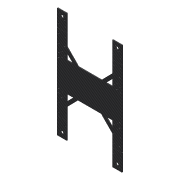
# Autodesk Inventor part: chassis mit motorlöcher
Saved by Autodesk Inventor 2018 (Build 220112000, 112)
## iProperties
Created: 2018-01-20
Part Number: chassis mit motorlöcher
Material: CFK
Document SubType Name: Modeling
Designer: fhinstall
Density: 1.43 g/cm^3
Appearance: Kohlenstofffaser
Mass: 133.015 g
Surface Area: 687.489 cm^2
Volume: 93.0173 cm^3
Author: fhinstall
Autodesk Inventor part; units mm, degrees
ref_plane "YZ Plane" through (0, 0, 0) normal (1, 0, 0) x (0, 1, 0)
ref_plane "XZ Plane" through (0, 0, 0) normal (0, 1, 0) x (-1, 0, 0)
ref_plane "XY Plane" through (0, 0, 0) normal (0, 0, 1) x (1, 0, 0)
sketch "Skizze1" plane through (0, 0, 0) normal (0, 1, 0) x (-1, 0, 0)
  line L0 (127.3199, 0) -> (-102.7808, 0) construction
  line L1 (0, 142.2638) -> (0, -235.5235) construction
  line L2 (100, 50) -> (100, 0)
  line L3 (70, 45) -> (0, 45)
  line L4 (0, 0) -> (100, 0)
  line L5 (0, 45) -> (0, 0)
  line L6 (100, 50) -> (100, 170)
  line L7 (100, 170) -> (70, 170)
  line L8 (70, 170) -> (70, 45)
  circle A0 centre (95, 41) radius 1.7
  line L9 (100, 140) -> (70, 140) construction
  circle A1 centre (85, 155) radius 4
  circle A2 centre (79.7789, 161.0614) radius 1.7
  circle A3 centre (92.1979, 161.2) radius 1.7
  circle A4 centre (90.2211, 148.9386) radius 1.7
  circle A5 centre (77.8021, 148.8) radius 1.7
  circle A6 centre (85, 155) radius 8 construction
  circle A7 centre (85, 155) radius 9.5 construction
  line L10 (79.7789, 161.0614) -> (90.2211, 148.9386) construction
  line L11 (92.1979, 161.2) -> (77.8021, 148.8) construction
  arc A8 (92.0223, 145.331) -> (96.9015, 153.9244) centre (85, 155) ccw construction
  line L12 (96.9015, 153.9244) -> (96.6242, 153.848) construction
  arc A9 (94.3917, 161.9459) -> (96.6242, 153.848) centre (95.508, 157.8969) ccw construction
  line L13 (94.3917, 161.9459) -> (94.669, 162.0223) construction
  arc A10 (94.669, 162.0223) -> (86.0756, 166.9015) centre (85, 155) ccw construction
  line L14 (86.0756, 166.9015) -> (86.152, 166.6242) construction
  arc A11 (78.0541, 164.3917) -> (86.152, 166.6242) centre (82.1031, 165.508) ccw construction
  line L15 (78.0541, 164.3917) -> (77.9777, 164.669) construction
  arc A12 (77.9777, 164.669) -> (73.0985, 156.0756) centre (85, 155) ccw construction
  line L16 (73.0985, 156.0756) -> (73.3758, 156.152) construction
  arc A13 (75.6083, 148.0541) -> (73.3758, 156.152) centre (74.492, 152.1031) ccw construction
  line L17 (75.6083, 148.0541) -> (75.331, 147.9777) construction
  arc A14 (75.331, 147.9777) -> (83.9244, 143.0985) centre (85, 155) ccw construction
  line L18 (83.9244, 143.0985) -> (83.848, 143.3758) construction
  arc A15 (91.9459, 145.6083) -> (83.848, 143.3758) centre (87.8969, 144.492) ccw construction
  line L19 (91.9459, 145.6083) -> (92.0223, 145.331) construction
  circle A16 centre (85, 155) radius 4 construction
  circle A17 centre (78.0432, 158.95) radius 1.25 construction
  circle A18 centre (89.6906, 163.2613) radius 1.25 construction
  circle A19 centre (91.9568, 151.05) radius 1.25 construction
  circle A20 centre (80.3094, 146.7387) radius 1.25 construction
  line L20 (70, 117.8095) -> (70, 117.3095)
  line L21 (100, 118) -> (70, 118)
  line L22 (70, 118) -> (70, 117.5)
  line L23 (70, 117.5) -> (100, 117.5)
  line L24 (100, 117.5) -> (100, 118)
  circle A21 centre (95.0005, 132.5) radius 1.7
  circle A22 centre (75.0005, 132.5) radius 1.7
  circle A23 centre (75, 105.2) radius 1.7
  circle A24 centre (95, 105.2) radius 1.7
  circle A25 centre (95, 79.2) radius 1.7
  circle A26 centre (75, 79.2) radius 1.7
  circle A27 centre (95.0005, 132.5) radius 1.7
  circle A28 centre (75.0005, 132.5) radius 1.7
  circle A29 centre (75, 105.2) radius 1.7
  circle A30 centre (95, 105.2) radius 1.7
  circle A31 centre (95, 79.2) radius 1.7
  circle A32 centre (75, 79.2) radius 1.7
  circle A33 centre (77, 54.3143) radius 1.7
  circle A34 centre (93, 54.3143) radius 1.7
  line L25 (70, 65) -> (70, 45)
  line L26 (70, 45) -> (50.4571, 45)
  line L27 (70, 65) -> (50.4571, 45)
  line L28 (70, 80) -> (35.8, 45)
  circle A35 centre (85, 61.7504) radius 1.7
  circle A36 centre (85, 45.7504) radius 1.7
  dimension "d75" = 19
  dimension "d10" = 100
  dimension "d12" = 30
  dimension "d13" = 170
  dimension "d14" = 45
  dimension "d22" = 5
  dimension "d23" = 4
  dimension "d26" = 3.4
  dimension "d59" = 30
  dimension "d60" = 8
  dimension "d61" = 15
  dimension "d64" = 3.4
  dimension "d65" = 3.4
  dimension "d66" = 3.4
  dimension "d67" = 3.4
  dimension "d70" = 7.8021
  dimension "d74" = 16
  dimension "d76" = 90
  dimension "d78" = 0.5
  dimension "d79" = 52
  dimension "d82" = 3.4
  dimension "d83" = 3.4
  dimension "d84" = 7
  dimension "d85" = 7
  dimension "d88" = 20
  dimension "d89" = 15
  dimension "d90" = 3.4
  dimension "d91" = 3.4
  dimension "d92" = 16
  constraints: 42 end point, 23 centre point, 14 point on line, 10 coincident, 7 perpendicular, 6 concentric, 3 midpoint, 3 parallel, 2 collinear, 2 horizontal, 2 point on circle, 2 vertical, 15 other
  measures "d10" distance between parallel lines of L1 L2
  measures "d12" distance of L6.end L7.end
  measures "d13" distance between parallel lines of L0 L7
  measures "d14" distance between parallel lines of L0 L3
  measures "d22" distance from line of L2 A0.centre
  measures "d23" distance from line of L3 A0.centre
  measures "d26" diameter of A0
  measures "d59" distance between parallel lines of L9 L7
  measures "d60" diameter of A1
  measures "d61" distance from line of L9 A1.centre
  measures "d64" diameter of A5
  measures "d65" diameter of A4
  measures "d66" diameter of A3
  measures "d67" diameter of A2
  measures "d70" distance from line of L6 L11.start
  measures "d74" diameter of A6
  measures "d76" angle of L10 L11
  measures "d78" distance of L22.end L21.end
  measures "d79" distance between parallel lines of L7 L21
  measures "d82" diameter of A33
  measures "d83" diameter of A34
  measures "d84" distance from line of L8 A33.centre
  measures "d85" distance from line of L6 A34.centre
  measures "d88" distance of L25.start L3.start
  measures "d89" distance of L25.start L28.start
  measures "d90" diameter of A35
  measures "d91" diameter of A36
  measures "d92" distance of A35.centre A36.centre
extrude "Extrusion1" add sketch "Skizze1" along normal blind 3 contours L2 L4 L5 L3 L8 L23 L6 | L21 L8 L7 L6 | L28 L8 L27 L3
ref_plane "Arbeitsebene1" through (0, 0, 45) normal (1, 0, 0) x (0, 1, 0)
ref_plane "Arbeitsebene2" through (0, 3, 0) normal (0, 0, -1) x (-1, 0, 0)
mirror "Spiegeln1" about plane through (0, 3, 0) normal (0, 0, -1) of "Extrusion1"
mirror "Spiegeln2" about plane through (0, 0, 45) normal (1, 0, 0) of "Extrusion1", "Spiegeln1"
